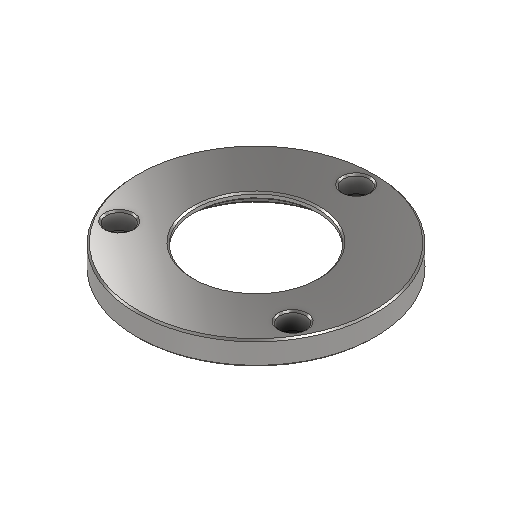
# Autodesk Inventor part: clamp_for_bearing
Saved by Autodesk Inventor 2026.2 (Build 302298000, 298)
## iProperties
Created: 2026-07-16
Part Number: clamp_for_bearing
Material: ステンレス鋼
Document SubType Name: Modeling
Designer: zetsu
Density: 8 g/cm^3
Appearance: 半つや出し
Author: zetsu
Autodesk Inventor part; units mm, degrees
ref_plane "YZ Plane" through (0, 0, 0) normal (1, 0, 0) x (0, 1, 0)
ref_plane "XZ Plane" through (0, 0, 0) normal (0, 1, 0) x (-1, 0, 0)
ref_plane "XY Plane" through (0, 0, 0) normal (0, 0, 1) x (1, 0, 0)
sketch "スケッチ1" plane through (0, 0, 0) normal (0, 1, 0) x (-1, 0, 0)
  circle A0 centre (0, 0) radius 37
  dimension "d0" = 74
  constraints: 1 centre point, 1 coincident
  measures "d0" diameter of A0
extrude "押し出し1" add sketch "スケッチ1" along normal blind 7.3
sketch "スケッチ2" plane through (0, 7.3, 0) normal (0, 1, 0) x (1, 0, 0)
  circle A0 centre (0, 0) radius 19
  dimension "d3" = 38
  constraints: 1 centre point, 1 coincident
  measures "d3" diameter of A0
extrude "押し出し2" cut sketch "スケッチ2" against normal through all
sketch "スケッチ3" plane through (0, 0, 0) normal (0, -1, 0) x (1, 0, 0)
  circle A0 centre (0, 0) radius 25.15
  dimension "d6" = 50.3
  constraints: 1 centre point, 1 coincident
  measures "d6" diameter of A0
extrude "押し出し3" cut sketch "スケッチ3" against normal blind 5.3
sketch "スケッチ6" plane through (0, 7.3, 0) normal (0, 1, 0) x (1, 0, 0)
  circle A0 centre (0, 31) radius 2.15
  circle A1 centre (-26.8468, -15.5) radius 2.15
  circle A2 centre (26.8468, -15.5) radius 2.15
  point P0 (0, 0)
  dimension "d21" = 4.3
  dimension "d22" = 31
  dimension "d25" = 360
  constraints: 3 centre point, 7 other
  measures "d21" diameter of A0
  measures "d22" distance of point (0, 0) A0.centre
extrude "押し出し6" cut sketch "スケッチ6" against normal through all
sketch "スケッチ7" plane through (0, 7.3, 0) normal (0, 1, 0) x (1, 0, 0)
  circle A0 centre (0, 31) radius 2.15 projected
  circle A1 centre (0, 31) radius 4
  circle A2 centre (-26.8468, -15.5) radius 4
  circle A3 centre (26.8468, -15.5) radius 4
  point P0 (0, 0)
  dimension "d29" = 8
  dimension "d32" = 360
  constraints: 3 centre point, 1 coincident, 7 other
  measures "d29" diameter of A1
extrude "押し出し7" cut sketch "スケッチ7" against normal blind 5.3 contours A0 | A1 | A2 | A3
chamfer "面取り1" distance 0.5 angle 45 8 edges at (37, 7.3, 0) (37, 0, 0) (-25.15, 0, 0) (-19, 7.3, 0) (-19, 5.3, 0) (22.8468, 7.3, 15.5) (-30.8468, 7.3, 15.5) (-4, 7.3, -31)
